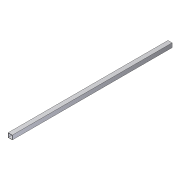
# Autodesk Inventor part: GE-12028-03
Saved by Autodesk Inventor 2012 (Build 160160000, 160)
## iProperties
Created: 2008-05-29
Part Number: GE-12028-03
Description: Support, Top and Bottom
Document SubType Name: Modeling
Designer: dfoster
Mass: 932.014 g
Surface Area: 5881.44 cm^2
Volume: 932.014 cm^3
Density: 1 g/cm^3
Material: Default
Author: narosenberg
Autodesk Inventor part; units mm, degrees
ref_plane "YZ Plane" through (0, 0, 0) normal (1, 0, 0) x (0, 1, 0)
ref_plane "XZ Plane" through (0, 0, 0) normal (0, 1, 0) x (-1, 0, 0)
ref_plane "XY Plane" through (0, 0, 0) normal (0, 0, 1) x (1, 0, 0)
sketch "Sketch1" plane through (0, 0, 0) normal (0, 0, 1) x (1, 0, 0)
  line L0 (-24.7686, 16.9571) -> (19.6814, 16.9571)
  line L1 (19.6814, 16.9571) -> (19.6814, -27.4929)
  line L2 (19.6814, -27.4929) -> (-24.7686, -27.4929)
  line L3 (-24.7686, -27.4929) -> (-24.7686, 16.9571)
  line L4 (-21.5936, 13.7821) -> (16.5064, 13.7821)
  line L5 (16.5064, 13.7821) -> (16.5064, -24.3179)
  line L6 (16.5064, -24.3179) -> (-21.5936, -24.3179)
  line L7 (-21.5936, -24.3179) -> (-21.5936, 13.7821)
  dimension "d0" = 44.45
  dimension "d1" = 44.45
  dimension "d2" = 3.175
  dimension "d3" = 3.175
  dimension "d4" = 3.175
  dimension "d5" = 3.175
  constraints: 16 end point, 4 parallel, 2 horizontal, 2 perpendicular
  measures "d0" distance of L0.start L0.end
  measures "d1" distance of L2.end L0.start
  measures "d2" distance between parallel lines of L1 L5
  measures "d3" distance between parallel lines of L0 L4
  measures "d4" distance between parallel lines of L3 L7
  measures "d5" distance between parallel lines of L2 L6
extrude "Extrusion1" add sketch "Sketch1" along normal blind 1701.8
equation "\"d1\" = d0"
equation "\"d3\" = d2"
equation "\"d4\" = d2"
equation "\"d5\" = d2"
body "Solid1"
